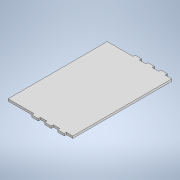
# Autodesk Inventor part: ramp2
Saved by Autodesk Inventor 2020 (Build 240168000, 168)
## iProperties
Created: 2019-11-21
Part Number: ramp2
Material: Generic
Document SubType Name: Modeling
Designer: shrey
Density: 1 g/cm^3
Appearance: Default
Author: shrey
Autodesk Inventor part; units mm, degrees
ref_plane "YZ Plane" through (0, 0, 0) normal (1, 0, 0) x (0, 1, 0)
ref_plane "XZ Plane" through (0, 0, 0) normal (0, 1, 0) x (-1, 0, 0)
ref_plane "XY Plane" through (0, 0, 0) normal (0, 0, 1) x (1, 0, 0)
sketch "Sketch1" plane through (0, 0, 0) normal (0, 1, 0) x (-1, 0, 0)
  line L0 (95.25, 146.05) -> (-95.25, 146.05)
  line L1 (-95.25, 146.05) -> (-95.25, -146.05)
  line L2 (-95.25, -146.05) -> (95.25, -146.05)
  line L3 (95.25, -146.05) -> (95.25, 146.05)
  line L4 (95.25, 146.05) -> (-95.25, -146.05) construction
  line L5 (-95.25, 146.05) -> (95.25, -146.05) construction
  line L6 (95.25, -146.05) -> (76.2, -146.05)
  line L7 (76.2, -146.05) -> (76.2, -152.4)
  line L8 (76.2, -152.4) -> (95.25, -152.4)
  line L9 (95.25, -152.4) -> (95.25, -146.05)
  line L10 (38.1, -146.05) -> (38.1, -152.4)
  line L11 (57.15, -146.05) -> (38.1, -146.05)
  line L12 (38.1, -152.4) -> (57.15, -152.4)
  line L13 (57.15, -152.4) -> (57.15, -146.05)
  line L14 (0, -146.05) -> (0, -152.4)
  line L15 (19.05, -146.05) -> (0, -146.05)
  line L16 (0, -152.4) -> (19.05, -152.4)
  line L17 (19.05, -152.4) -> (19.05, -146.05)
  line L18 (-38.1, -146.05) -> (-38.1, -152.4)
  line L19 (-19.05, -146.05) -> (-38.1, -146.05)
  line L20 (-38.1, -152.4) -> (-19.05, -152.4)
  line L21 (-19.05, -152.4) -> (-19.05, -146.05)
  line L22 (-76.2, -146.05) -> (-76.2, -152.4)
  line L23 (-57.15, -146.05) -> (-76.2, -146.05)
  line L24 (-76.2, -152.4) -> (-57.15, -152.4)
  line L25 (-57.15, -152.4) -> (-57.15, -146.05)
  line L26 (95.25, 0) -> (-95.25, 0) construction
  line L27 (95.25, 146.05) -> (76.2, 146.05)
  line L28 (76.2, 146.05) -> (76.2, 152.4)
  line L29 (76.2, 152.4) -> (95.25, 152.4)
  line L30 (95.25, 152.4) -> (95.25, 146.05)
  line L31 (57.15, 146.05) -> (38.1, 146.05)
  line L32 (38.1, 146.05) -> (38.1, 152.4)
  line L33 (38.1, 152.4) -> (57.15, 152.4)
  line L34 (57.15, 152.4) -> (57.15, 146.05)
  line L35 (19.05, 146.05) -> (0, 146.05)
  line L36 (0, 146.05) -> (0, 152.4)
  line L37 (0, 152.4) -> (19.05, 152.4)
  line L38 (19.05, 152.4) -> (19.05, 146.05)
  line L39 (-19.05, 146.05) -> (-38.1, 146.05)
  line L40 (-38.1, 146.05) -> (-38.1, 152.4)
  line L41 (-38.1, 152.4) -> (-19.05, 152.4)
  line L42 (-19.05, 152.4) -> (-19.05, 146.05)
  line L43 (-57.15, 146.05) -> (-76.2, 146.05)
  line L44 (-76.2, 146.05) -> (-76.2, 152.4)
  line L45 (-76.2, 152.4) -> (-57.15, 152.4)
  line L46 (-57.15, 152.4) -> (-57.15, 146.05)
  point P0 (0, 0)
  dimension "d0" = 292.1
  dimension "d1" = 190.5
  dimension "d2" = 19.05
  dimension "d3" = 6.35
  dimension "d6" = 38.1
  dimension "d11" = 19.05
  dimension "d12" = 6.35
  dimension "d15" = 38.1
  constraints: 94 end point, 6 parallel, 5 horizontal, 4 midpoint, 3 perpendicular, 64 other
  measures "d0" distance of L0.end L1.end
  measures "d1" distance of L0.start L0.end
  measures "d2" distance of L8.end L7.end
  measures "d3" distance of L7.end L6.end
  measures "d6" distance of L6.end L10.start
  measures "d11" distance of L28.end L29.end
  measures "d12" distance of L29.end L0.start
  measures "d15" distance of L0.start L31.start
extrude "Extrusion2" add sketch "Sketch1" along normal blind 6.35 contours L3 L2 L1 L0 | L0 L36 L37 L38 | L17 L16 L14 L2 | L0 L40 L41 L42 | L21 L20 L18 L2 | L0 L44 L45 L46 | L25 L24 L22 L2
body "Solid2"
